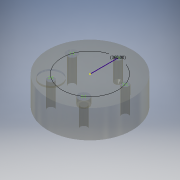
# Autodesk Inventor part: Drilled Holes
Saved by Autodesk Inventor 2018 (Build 220112000, 112)
## iProperties
Created: 2005-07-06
Part Number: Drilled Holes
Document SubType Name: Modeling
Designer: Administrator
Manufacturer: Standard
Standards Organization: Custom
Material: Generic
Density: 1 g/cm^3
Appearance: Lexan (Smoked)
Author: Administrator
Autodesk Inventor part; units mm, degrees
ref_plane "YZ Plane" through (0, 0, 0) normal (1, 0, 0) x (0, 1, 0)
ref_plane "XZ Plane" through (0, 0, 0) normal (0, 1, 0) x (-1, 0, 0)
ref_plane "XY Plane" through (0, 0, 0) normal (0, 0, 1) x (1, 0, 0)
sketch "Sketch1" plane through (0, 0, 0) normal (0, 0, 1) x (1, 0, 0)
  circle A0 centre (0, 0) radius 38.1
  dimension "d0" = 76.2
  constraints: 1 centre point
  measures "d0" diameter of A0
extrude "Extrusion1" add sketch "Sketch1" against normal blind 25.4
sketch "Sketch2" plane through (0, 0, 0) normal (0, 0, 1) x (1, 0, 0)
  line L0 (0, 0) -> (0, 25.4)
  point P0 (-24.1568, 7.849)
  point P1 (-14.9297, -20.549)
  point P2 (14.9297, -20.549)
  point P3 (24.1568, 7.849)
  dimension "d5" = 360
  constraints: 2 end point, 1 vertical, 6 other
hole "Hole1" at (0, 25.4, 0) direction (0, 0, -1) diameter 6.35 depth 19.05 tip angle 118
sketch "Sketch3" plane through (0, 0, 0) normal (0, 0, 1) x (1, 0, 0)
  point P0 (0, 0)
sketch "Sketch4" plane through (0, 0, 0) normal (0, 0, 1) x (1, 0, 0)
  point P0 (0, 0)
sketch "Sketch5" plane through (0, 0, 0) normal (0, 0, 1) x (1, 0, 0)
  point P0 (0, 0)
sketch "Sketch6" plane through (0, 0, 0) normal (0, 0, 1) x (1, 0, 0)
  point P0 (0, 0)
sketch "Sketch7" plane through (0, 0, 0) normal (0, 0, 1) x (1, 0, 0)
  point P0 (0, 0)
hole "Hole2" at (24.1568, 7.849, 0) direction (0, 0, -1) diameter 6.35 end through all
hole "Hole3" at (14.9297, -20.549, 0) direction (0, 0, -1) diameter 6.35 end through all counterbore diameter 9.525 counterbore depth 6.35
hole "Hole4" at (-14.9297, -20.549, 0) direction (0, 0, -1) diameter 6.35 end through all counterbore diameter 19.05 counterbore depth 1.5875
hole "Hole5" at (-24.1568, 7.849, 0) direction (0, 0, -1) diameter 6.35 end through all countersink diameter 9.525 countersink angle 82
body "Solid1"
